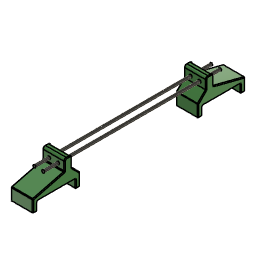
Bracket aquario v2 (Autodesk Fusion 360 design; units mm, degrees)
Autodesk Fusion 360 part; units mm, degrees
sketch "Sketch1" plane through (0, 0, 0) normal (1, 0, 0) x (0, 1, 0)
  line L0 (0, 0) -> (0, 12)
  line L1 (0, 12) -> (52, 12)
  line L2 (52, 12) -> (52, 0)
  line L3 (52, 0) -> (58, 0)
  line L4 (58, 0) -> (58, 17)
  line L5 (58, 17) -> (47, 28)
  line L6 (47, 28) -> (47, 43)
  line L7 (47, 43) -> (37, 43)
  line L8 (37, 43) -> (37, 28)
  line L9 (37, 28) -> (-6, 17)
  line L10 (-6, 17) -> (-6, 0)
  line L11 (-6, 0) -> (0, 0)
  dimension "d1" = 10
  dimension "d2" = 6
  dimension "d3" = 52
  dimension "d4" = 15
  dimension "d5" = 12
  dimension "d6" = 5
  dimension "d7" = 135
  dimension "d8" = 5
  constraint coincident L0.start L11.end
  constraint vertical L0
  constraint perpendicular L0 L1
  constraint perpendicular L1 L2
  constraint perpendicular L2 L3
  constraint perpendicular L1 L4
  constraint perpendicular L4 L7
  constraint perpendicular L7 L8
  constraint perpendicular L7 L10
  constraint perpendicular L0 L11
  constraint vertical L6
  constraint equal L3 L11
  constraint equal L4 L10
  constraint equal L6 L8
  constraint collinear L3 L11
  measures "d1" distance of L6.end L7.end
  measures "d2" distance of L10.end L0.start
  measures "d3" distance of L0.end L1.end
  measures "d4" distance of L7.end L8.end
  measures "d5" distance of L0.start L0.end
  measures "d6" distance of L1 L4.end
  measures "d7" angle of L4 L5
  measures "d8" horizontal distance of L1.end L5.end
extrude "Extrude1" add sketch "Sketch1" along normal blind 30 makes body 1
fillet "Fillet1" radius 1 9 edges at (15, 0, 12) (15, -6, 17) (15, -6, 0) (15, 0, 0) (15, 52, 12) (15, 58, 17) (15, 37, 28) (15, 52, 0) (15, 58, 0) on bodies 1
fillet "Fillet2" radius 3 2 edges at (15, 37, 43) (15, 47, 43) on bodies 1
chamfer "Chamfer1" distance 1 angle 45 46 edges at (30, 15.5, 22.5) (30, -5.7899, 16.8369) (30, -6, 8.6118) (30, -5.7071, 0.2929) (30, -3, 0) (30, -0.2929, 0.2929) (30, 0, 6) (30, 0.2929, 11.7071) (30, 26, 12) (30, 51.7071, 11.7071) (30, 52, 6) (30, 52.2929, 0.2929) (30, 55, 0) (30, 57.7071, 0.2929) (30, 58, 8.7929) (30, 57.9239, 16.9685) (30, 52.3536, 22.6464) (30, 47, 34) (30, 46.1213, 42.1213) (30, 42, 43) (30, 37.8787, 42.1213) (30, 37, 34.3882) (30, 36.7899, 28.1631) (0, 15.5, 22.5) (0, -5.7899, 16.8369) (0, -6, 8.6118) (0, -5.7071, 0.2929) (0, -3, 0) (0, -0.2929, 0.2929) (0, 0, 6) (0, 0.2929, 11.7071) (0, 26, 12) (0, 51.7071, 11.7071) (0, 52, 6) (0, 52.2929, 0.2929) (0, 55, 0) (0, 57.7071, 0.2929) (0, 58, 8.7929) (0, 57.9239, 16.9685) (0, 52.3536, 22.6464) (0, 47, 34) (0, 46.1213, 42.1213) (0, 42, 43) (0, 37.8787, 42.1213) (0, 37, 34.3882) (0, 36.7899, 28.1631) on bodies 1
sketch "Sketch2" plane through (0, 47, 0) normal (0, 1, 0) x (-1, 0, 0)
  line L0 (-1, 28) -> (-1, 40)
  line L1 (-1, 40) -> (-29, 40)
  line L2 (-29, 40) -> (-29, 28)
  line L3 (-29, 28) -> (-1, 28)
  circle A0 centre (-9, 34) radius 2.05
  line L4 (-29, 34) -> (-1, 34) construction
  circle A1 centre (-21, 34) radius 2.05
  line L5 (-15, 34) -> (-15, 40) construction
  dimension "d16" = 4.1
  dimension "d17" = 12
  constraint midpoint L2 L4.start
  constraint midpoint L0 L4.end
  constraint coincident A0.centre L4
  constraint coincident L4 A1.centre
  constraint equal A0 A1
  constraint midpoint L4 L5.start
  constraint midpoint L1 L5.end
  constraint symmetric A0 A1 L5
  measures "d16" diameter of A0
  measures "d17" distance of A0.centre A1.centre
extrude "Extrude2" cut sketch "Sketch2" against normal blind 18 contours A0 | A1 bodies 1
ref_plane "WorkPlane1" through (15, 138, 8.7929) normal (0, 1, 0) x (0, 0, 1)
mirror "Mirror1" about plane through (15, 138, 8.7929) normal (0, 1, 0) of bodies 1 makes body 2
sketch "Sketch3" plane through (0, 37, 0) normal (0, -1, 0) x (1, 0, 0)
  circle A0 centre (21, 34) radius 2.05
  circle A1 centre (9, 34) radius 2.05
  line L0 (1, 40) -> (1, 28.7764)
  line L1 (1, 28.7764) -> (29, 28.7764)
  line L2 (29, 28.7764) -> (29, 40)
  line L3 (29, 40) -> (1, 40)
  circle A2 centre (9, 34) radius 2
  circle A3 centre (21, 34) radius 2
  dimension "d23" = 4
  dimension "d24" = 4
  constraint concentric A1 A2
  constraint concentric A0 A3
  measures "d23" diameter of A2
  measures "d24" diameter of A3
extrude "Extrude3" add sketch "Sketch3" along normal blind 20 and the other way blind 220 separate body contours A2 | A3 makes body 3 at (10.9171, 183.6667, 33.4302) makes body 4 at (22.7498, 183.6667, 34.9686)
